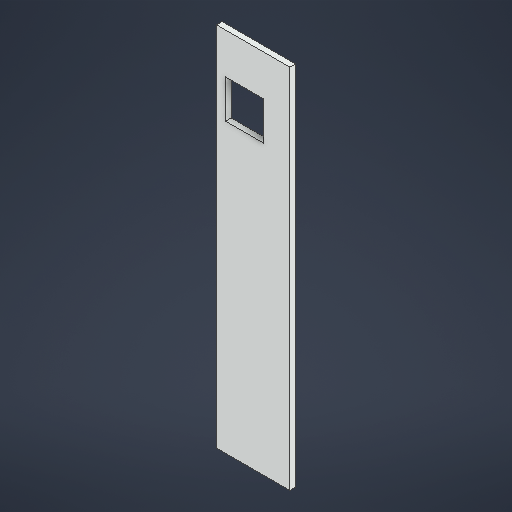
# Autodesk Inventor part: partttt
Saved by Autodesk Inventor 2026.2 (Build 302298010, 298A)
## iProperties
Created: 2026-03-03
Part Number: partttt
Material: Generic
Document SubType Name: Modeling
Designer: shahd
Density: 1 g/cm^3
Appearance: Default
Mass: 75.5208 g
Surface Area: 346.403 cm^2
Volume: 75.5208 cm^3
Author: shahd
Autodesk Inventor part; units mm, degrees
ref_plane "YZ Plane" through (0, 0, 0) normal (1, 0, 0) x (0, 1, 0)
ref_plane "XZ Plane" through (0, 0, 0) normal (0, 1, 0) x (-1, 0, 0)
ref_plane "XY Plane" through (0, 0, 0) normal (0, 0, 1) x (1, 0, 0)
sketch "Sketch1" plane through (0, 0, 0) normal (0, 0, 1) x (1, 0, 0)
  line L0 (0, 0) -> (65, 0)
  line L1 (65, 0) -> (65, 325.203)
  line L2 (65, 325.203) -> (0, 325.203)
  line L3 (0, 325.203) -> (0, 0)
  line L4 (8, 289.203) -> (42, 289.203)
  line L5 (42, 289.203) -> (42, 255.203)
  line L6 (42, 255.203) -> (8, 255.203)
  line L7 (8, 255.203) -> (8, 289.203)
  point P0 (32.5, 325.203)
  dimension "d0" = 65
  dimension "d1" = 325.203
  dimension "d8" = 34
  dimension "d9" = 34
  dimension "d10" = 8
  dimension "d11" = 36
  constraints: 16 end point, 4 parallel, 2 horizontal, 2 perpendicular, 1 coincident, 1 midpoint
  measures "d0" distance of L2.end L1.end
  measures "d1" distance of L1.end L0.end
  measures "d8" distance of L4.start L4.end
  measures "d9" distance of L6.end L4.start
  measures "d10" distance between parallel lines of L3 L7
  measures "d11" distance from line of point (32.5, 325.203) L4
extrude "Extrusion1" add sketch "Sketch1" along normal blind 5
body "Solid1"
